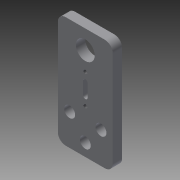
# Autodesk Inventor part: Plaque support
Saved by Autodesk Inventor 2015 SP1 (Build 190203100, 203)
## iProperties
Created: 2015-04-11
Part Number: Plaque support
Material: Generic
Document SubType Name: Modeling
Designer: Cyril
Density: 1 g/cm^3
Appearance: Default
Author: Cyril
Autodesk Inventor part; units mm, degrees
ref_plane "YZ Plane" through (0, 0, 0) normal (1, 0, 0) x (0, 1, 0)
ref_plane "XZ Plane" through (0, 0, 0) normal (0, 1, 0) x (-1, 0, 0)
ref_plane "XY Plane" through (0, 0, 0) normal (0, 0, 1) x (1, 0, 0)
sketch "Sketch1" plane through (0, 0, 0) normal (0, 0, 1) x (1, 0, 0)
  line L0 (-17.5, 35.5) -> (17.5, 35.5)
  line L1 (17.5, 35.5) -> (17.5, -35.5)
  line L2 (17.5, -35.5) -> (-17.5, -35.5)
  line L3 (-17.5, -35.5) -> (-17.5, 35.5)
  line L4 (-17.5, 35.5) -> (17.5, -35.5) construction
  line L5 (17.5, 35.5) -> (-17.5, -35.5) construction
  circle A0 centre (-10, -15.5) radius 3.5
  circle A1 centre (0, -27.5) radius 3.5
  circle A2 centre (10, -15.5) radius 3.5
  circle A3 centre (0, 23.5) radius 6
  line L6 (0, 35.5) -> (0, -35.5) construction
  line L7 (0, 6) -> (0, -2) construction
  line L8 (-1.5, 6) -> (-1.5, -2)
  line L9 (1.5, -2) -> (1.5, 6)
  arc A4 (1.5, 6) -> (-1.5, 6) centre (0, 6) ccw
  arc A5 (-1.5, -2) -> (1.5, -2) centre (0, -2) ccw
  line L10 (-1.5, 2) -> (1.5, 2) construction
  point P0 (0, 0)
  point P1 (0, 2)
  point P2 (0, 11.5)
  point P3 (0, -7.5)
  dimension "d3" = 35
  dimension "d4" = 7
  dimension "d6" = 7
  dimension "d7" = 7
  dimension "d12" = 12
  dimension "d13" = 12
  dimension "d36" = 1.5
  dimension "d37" = 8
  dimension "d38" = 19
  dimension "d39" = 12
  dimension "d40" = 12
  dimension "d41" = 8
  dimension "d42" = 8
  dimension "d43" = 20
  constraints: 24 end point, 7 midpoint, 6 centre point, 6 point on line, 4 point on circle, 4 tangent, 3 parallel, 2 symmetric about line, 1 horizontal, 1 horizontal alignment, 1 perpendicular
  measures "d3" distance of L0.start L0.end
  measures "d4" diameter of A0
  measures "d6" diameter of A2
  measures "d7" diameter of A1
  measures "d12" diameter of A3
  measures "d13" distance from line of L0 A3.centre
  measures "d36" radius of A4
  measures "d37" distance of L7.end L7.start
  measures "d38" distance of point (0, -7.5) point (0, 11.5)
  measures "d39" distance of point (0, 11.5) A3.centre
  measures "d40" vertical distance of A1.centre A0.centre
  measures "d41" distance from line of L2 A1.centre
  measures "d42" vertical distance of A0.centre point (0, -7.5)
  measures "d43" distance of A2.centre A0.centre
extrude "Extrusion4" add sketch "Sketch1" along normal blind 6
hole "Hole1" at (0, -7.5, 0) at (0, 11.5, 0) direction (0, 0, 1) diameter 2.459 depth 8.8 tip angle 118 thread size "M3x0.5" class "6H" standard "ANSI Metric M Profile"
fillet "Fillet3" radius 5 4 edges at (-17.5, 35.5, 3) (17.5, 35.5, 3) (-17.5, -35.5, 3) (17.5, -35.5, 3)
equation "\"d6\" = d4"
equation "\"d7\" = d4"
body "Solid3"
